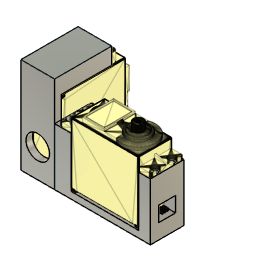
TARO2_arm_upper v1 (Autodesk Fusion 360 design; units mm, degrees)
Autodesk Fusion 360 part; units mm, degrees
sketch "スケッチ1" plane through (0, 0, 0) normal (0, 0, 1) x (1, 0, 0)
  line L0 (0, 0) -> (-34.35, 0)
  line L1 (-34.35, 0) -> (-34.35, 9.85)
  line L2 (-34.35, 9.85) -> (0, 9.85)
  line L3 (0, 9.85) -> (0, 0)
  line L4 (0, 0) -> (-24.35, 0)
  line L5 (-24.35, 0) -> (-24.35, -9.85)
  line L6 (-24.35, -9.85) -> (0, -9.85)
  line L7 (0, -9.85) -> (0, 0)
  line L8 (-34.35, 9.85) -> (14.25, 9.85)
  line L9 (14.25, 9.85) -> (14.25, -10)
  line L10 (14.25, -10) -> (-34.35, -10)
  line L11 (-34.35, -10) -> (-34.35, 9.85)
  line L12 (0, 0) -> (-34.35, 0)
  line L13 (14.25, -10) -> (-34.35, -10)
  line L14 (-34.35, 0) -> (-34.35, 9.85)
  line L15 (14.25, 9.85) -> (14.25, -10)
  line L16 (-34.35, 9.85) -> (14.25, 9.85)
  line L17 (0, 0) -> (-24.35, 0)
  line L18 (0, -9.85) -> (0, 0)
  line L19 (-24.35, 0) -> (-24.35, -9.85)
  line L20 (0, 9.85) -> (0, 0)
  line L21 (-34.35, -10) -> (-34.35, 9.85)
  line L22 (-24.35, -9.85) -> (0, -9.85)
  line L23 (-34.35, 9.85) -> (0, 9.85)
  dimension "d2" = 34.35
  dimension "d3" = 9.85
  dimension "d4" = 9.85
  dimension "d5" = 48.6
  dimension "d6" = 34.35
  dimension "d7" = 9.85
  dimension "d8" = 9.85
  dimension "d9" = 48.6
  constraint horizontal L0
  constraint vertical L1
  constraint horizontal L2
  constraint vertical L3
  constraint horizontal L4
  constraint vertical L5
  constraint horizontal L6
  constraint vertical L7
  constraint horizontal L8
  constraint vertical L9
  constraint horizontal L10
  constraint vertical L11
  constraint horizontal L12
  constraint vertical L14
  constraint horizontal L23
  constraint vertical L20
  constraint horizontal L17
  constraint vertical L19
  constraint horizontal L22
  constraint vertical L18
  constraint horizontal L16
  constraint vertical L15
  constraint horizontal L13
  constraint vertical L21
  measures "d2" distance of L0.start L0.end
  measures "d3" distance of L0.start L2.end
  measures "d4" distance of L0.start L6.end
  measures "d5" distance of L1.end L8.end
  measures "d6" distance of L0.start L0.end
  measures "d7" distance of L0.start L2.end
  measures "d8" distance of L0.start L6.end
  measures "d9" distance of L1.end L8.end
other "基準メッシュ フィーチャ1" in component "MG996R bracket(bairing) v1"
other "修正1" in component "MG996R bracket(bairing) v1"
other "修正2" in component "MG996R bracket(bairing) v1"
sketch "スケッチ1 (2)" plane through (0, 0, 0) normal (0, 0, 1) x (1, 0, 0) in component "MG996R bracket(bairing) v1"
other "修正3" in component "MG996R bracket(bairing) v1"
sketch "スケッチ2" plane through (0, 0, 0) normal (0, 0, 1) x (1, 0, 0) in component "MG996R bracket(bairing) v1"
  line L0 (-20, 10) -> (20, 10)
  line L1 (20, 10) -> (20, -10)
  line L2 (20, -10) -> (-20, -10)
  line L3 (-20, -10) -> (-20, 10)
  line L4 (-20, 10) -> (20, -10) construction
  line L5 (20, 10) -> (-20, -10) construction
  line L6 (20, -10) -> (27, -10)
  line L7 (27, -10) -> (27, 10)
  line L8 (27, 10) -> (20, 10)
  line L9 (20, 10) -> (20, -10)
  line L10 (-20, -10) -> (-27, -10)
  line L11 (-27, -10) -> (-27, 10)
  line L12 (-27, 10) -> (-20, 10)
  line L13 (-20, 10) -> (-20, -10)
  dimension "d1" = 7
  dimension "d2_1" = 20
  dimension "d3_1" = 7
  dimension "d4_1" = 20
  constraint horizontal L0
  constraint perpendicular L0 L1
  constraint parallel L0 L2
  constraint parallel L1 L3
  constraint coincident L4 origin
  constraint coincident L5 origin
  constraint horizontal L6
  constraint vertical L7
  constraint horizontal L8
  constraint vertical L9
  constraint horizontal L10
  constraint vertical L11
  constraint horizontal L12
  constraint vertical L13
  measures "d1" distance of L1.end L6.end
  measures "d2_1" distance of L1.end L0.end
  measures "d3_1" distance of L2.end L10.end
  measures "d4_1" distance of L2.end L0.start
extrude "押し出し1" add sketch "スケッチ2" along normal blind 3 makes body 1 in component "MG996R bracket(bairing) v1"
sketch "スケッチ3" plane through (0, 0, 3) normal (0, 0, 1) x (-1, 0, 0) in component "MG996R bracket(bairing) v1"
  line L0 (27, 10) -> (-27, 10)
  line L1 (-27, 10) -> (-27, -10)
  line L2 (-27, -10) -> (27, -10)
  line L3 (27, -10) -> (27, 10)
  line L4 (27, 10) -> (20, 10)
  line L5 (20, 10) -> (20, -10)
  line L6 (20, -10) -> (27, -10)
  line L7 (27, -10) -> (27, 10)
  line L8 (-27, 10) -> (-20, 10)
  line L9 (-20, 10) -> (-20, -10)
  line L10 (-20, -10) -> (-27, -10)
  line L11 (-27, -10) -> (-27, 10)
  constraint horizontal L4
  constraint vertical L5
  constraint horizontal L6
  constraint vertical L7
  constraint coincident L2 L5.end
  constraint coincident L0.start L3.end
  constraint horizontal L8
  constraint vertical L9
  constraint horizontal L10
  constraint vertical L11
  constraint coincident L0.end L1.start
extrude "押し出し2" add sketch "スケッチ3" along normal blind 5 contours L0 L2 L3 L4 L5 L6 L7 | L0 L1 L2 L8 L9 L10 L11 bodies 1 in component "MG996R bracket(bairing) v1"
sketch "スケッチ4" plane through (0, 0, 8) normal (0, 0, 1) x (-1, 0, 0) in component "MG996R bracket(bairing) v1"
  line L0 (-27, -10) -> (-20, -10)
  line L1 (-20, -10) -> (-20, 10)
  line L2 (-20, 10) -> (-27, 10)
  line L3 (-27, 10) -> (-27, -10)
  line L4 (-20, 10) -> (-27, 10)
  line L5 (-27, 10) -> (-27, 5)
  line L6 (-27, 5) -> (-20, 5)
  line L7 (-20, 5) -> (-20, 10)
  line L8 (-27, -10) -> (-20, -10)
  line L9 (-20, -10) -> (-20, -5)
  line L10 (-20, -5) -> (-27, -5)
  line L11 (-27, -5) -> (-27, -10)
  dimension "d9_1" = 7
  dimension "d10" = 5
  constraint horizontal L4
  constraint vertical L5
  constraint horizontal L6
  constraint vertical L7
  constraint coincident L3 L5.end
  constraint coincident L1.end L2.start
  constraint horizontal L8
  constraint vertical L9
  constraint horizontal L10
  constraint vertical L11
  constraint coincident L0.start L3.end
  measures "d9_1" distance of L0.start L0.end
  measures "d10" distance of L0.start L10.end
extrude "押し出し3" add sketch "スケッチ4" along normal blind 9 contours L0 L1 L3 L8 L9 L10 L11 | L1 L2 L3 L4 L5 L6 L7 bodies 1 in component "MG996R bracket(bairing) v1"
sketch "スケッチ5" plane through (0, 0, 17) normal (0, 0, 1) x (-1, 0, 0) in component "MG996R bracket(bairing) v1"
  line L0 (-27, -5) -> (-27, -10)
  line L1 (-27, -10) -> (-20, -10)
  line L2 (-20, -10) -> (-20, -5)
  line L3 (-20, -5) -> (-27, -5)
  line L4 (-20, 10) -> (-27, 10)
  line L5 (-27, 10) -> (-27, -10)
  line L6 (-27, -10) -> (-20, -10)
  line L7 (-20, -10) -> (-20, 10)
  constraint horizontal L4
  constraint vertical L5
  constraint horizontal L6
  constraint vertical L7
  constraint coincident L0.end L1.start
extrude "押し出し4" add sketch "スケッチ5" along normal blind 16 bodies 1 in component "MG996R bracket(bairing) v1"
extrude "押し出し5" add 1 faces at (-22.3333, 3.3333, 8) along direction (0, 0, 1) blind 25 on bodies 1 bodies 1 in component "MG996R bracket(bairing) v1"
sketch "スケッチ6" plane through (0, 0, 33) normal (0, 0, 1) x (-1, 0, 0) in component "MG996R bracket(bairing) v1"
  line L0 (-20, -10) -> (-20, 10)
  line L1 (-20, 10) -> (-27, 10)
  line L2 (-27, 10) -> (-27, -10)
  line L3 (-27, -10) -> (-20, -10)
  circle A0 centre (-25, 5) radius 1.5
  circle A1 centre (-25, -5) radius 1.5
  circle A2 centre (24.95, 5.2) radius 1.5
  circle A3 centre (25, -4.8) radius 1.5
  dimension "d17" = 3
  dimension "d18" = 3
  dimension "d19" = 3
  dimension "d20" = 3
  measures "d17" diameter of A0
  measures "d18" diameter of A1
  measures "d19" diameter of A2
  measures "d20" diameter of A3
extrude "押し出し6" cut sketch "スケッチ6" against normal blind 5 contours A0 | A1 | A2 | A3 bodies 1 in component "MG996R bracket(bairing) v1"
thread "ねじ1" "ISO Metric profile 3.0 M3x0.5 M3x0.5 6H" major diameter 3.086 minor diameter 2.529 pitch 0.5 angle 60 resizes the face on face at (-26.4981, 4.8748, 29.6667) on bodies 1 in component "MG996R bracket(bairing) v1"
thread "ねじ2" "ISO Metric profile 3.0 M3x0.5 M3x0.5 6H" major diameter 3.086 minor diameter 2.529 pitch 0.5 angle 60 resizes the face on face at (-26.4481, -5.1252, 29.6667) on bodies 1 in component "MG996R bracket(bairing) v1"
thread "ねじ3" "ISO Metric profile 3.0 M3x0.5 M3x0.5 6H" major diameter 3.086 minor diameter 2.529 pitch 0.5 angle 60 resizes the face on face at (23.5019, -4.9252, 29.6667) on face at (23.5019, 5.0748, 29.6667) on bodies 1 in component "MG996R bracket(bairing) v1"
extrude "押し出し7" add 1 faces at (-9, -3.3333, 0) along direction (0, 0, -1) blind 1 on bodies 1 bodies 1 in component "MG996R bracket(bairing) v1"
sketch "スケッチ7" plane through (0, 0, 0) normal (0, 0, 1) x (1, 0, 0) in component "MG996R bracket(bairing) v1"
  line L0 (-20, -10) -> (10.1, -10)
  line L1 (10.1, -10) -> (10.1, 10)
  line L2 (10.1, 10) -> (-20, 10)
  line L3 (-20, 10) -> (-20, -10)
  circle A0 centre (10.1, 0) radius 7
  dimension "d31" = 30.1
  dimension "d32" = 14
  constraint horizontal L0
  constraint vertical L1
  constraint horizontal L2
  constraint vertical L3
  constraint midpoint L1 A0.centre
  measures "d31" distance of L0.start L0.end
  measures "d32" diameter of A0
move_body "移動1" bodies 1 to x (1, 0, 0) y (0, 1, 0) z (0, 0, 1) at (0, 0, 1) in component "MG996R bracket(bairing) v1"
other "修正4" in component "MG996R bracket(bairing) v1"
extrude "押し出し8" cut sketch "スケッチ7" along normal blind 4 contours L1 A0 | L1 A0 bodies 1 in component "MG996R bracket(bairing) v1"
extrude "押し出し9" add 1 faces at (-27, -3.3333, 11.3333) along direction (-1, 0, 0) blind 3 on bodies 1 bodies 1 in component "MG996R bracket(bairing) v1"
sketch "スケッチ8" plane through (-30, 0, 0) normal (-1, 0, 0) x (0, -1, 0) in component "MG996R bracket(bairing) v1"
  line L0 (10, 0) -> (10, 34)
  line L1 (10, 34) -> (-10, 34)
  line L2 (-10, 34) -> (-10, 0)
  line L3 (-10, 0) -> (10, 0)
other "基準メッシュ フィーチャ1'" in component "MG996R bracket(bairing) v1 (1)"
other "修正1'" in component "MG996R bracket(bairing) v1 (1)"
other "修正2'" in component "MG996R bracket(bairing) v1 (1)"
sketch "スケッチ1 (3)" plane through (0, 0, 0) normal (0, 0, 1) x (1, 0, 0) in component "MG996R bracket(bairing) v1 (1)"
other "修正3'" in component "MG996R bracket(bairing) v1 (1)"
sketch "スケッチ2 (2)" plane through (0, 0, 0) normal (0, 0, 1) x (1, 0, 0) in component "MG996R bracket(bairing) v1 (1)"
  line L0 (-20, 10) -> (20, 10)
  line L1 (20, 10) -> (20, -10)
  line L2 (20, -10) -> (-20, -10)
  line L3 (-20, -10) -> (-20, 10)
  line L4 (-20, 10) -> (20, -10) construction
  line L5 (20, 10) -> (-20, -10) construction
  line L6 (20, -10) -> (27, -10)
  line L7 (27, -10) -> (27, 10)
  line L8 (27, 10) -> (20, 10)
  line L9 (20, 10) -> (20, -10)
  line L10 (-20, -10) -> (-27, -10)
  line L11 (-27, -10) -> (-27, 10)
  line L12 (-27, 10) -> (-20, 10)
  line L13 (-20, 10) -> (-20, -10)
  dimension "d1_1" = 7
  dimension "d2_2" = 20
  dimension "d3_2" = 7
  dimension "d4_2" = 20
  constraint horizontal L0
  constraint perpendicular L0 L1
  constraint parallel L0 L2
  constraint parallel L1 L3
  constraint coincident L4 origin
  constraint coincident L5 origin
  constraint horizontal L6
  constraint vertical L7
  constraint horizontal L8
  constraint vertical L9
  constraint horizontal L10
  constraint vertical L11
  constraint horizontal L12
  constraint vertical L13
  measures "d1_1" distance of L1.end L6.end
  measures "d2_2" distance of L1.end L0.end
  measures "d3_2" distance of L2.end L10.end
  measures "d4_2" distance of L2.end L0.start
extrude "押し出し1'" add sketch "スケッチ2 (2)" along normal blind 3 separate body makes body 2 in component "MG996R bracket(bairing) v1 (1)"
sketch "スケッチ3 (2)" plane through (0, 0, 3) normal (0, 0, 1) x (-1, 0, 0) in component "MG996R bracket(bairing) v1 (1)"
  line L0 (27, 10) -> (-27, 10)
  line L1 (-27, 10) -> (-27, -10)
  line L2 (-27, -10) -> (27, -10)
  line L3 (27, -10) -> (27, 10)
  line L4 (27, 10) -> (20, 10)
  line L5 (20, 10) -> (20, -10)
  line L6 (20, -10) -> (27, -10)
  line L7 (27, -10) -> (27, 10)
  line L8 (-27, 10) -> (-20, 10)
  line L9 (-20, 10) -> (-20, -10)
  line L10 (-20, -10) -> (-27, -10)
  line L11 (-27, -10) -> (-27, 10)
  constraint horizontal L4
  constraint vertical L5
  constraint horizontal L6
  constraint vertical L7
  constraint coincident L2 L5.end
  constraint coincident L0.start L3.end
  constraint horizontal L8
  constraint vertical L9
  constraint horizontal L10
  constraint vertical L11
  constraint coincident L0.end L1.start
extrude "押し出し2'" add sketch "スケッチ3 (2)" along normal blind 5 contours L0 L2 L3 L4 L5 L6 L7 | L0 L1 L2 L8 L9 L10 L11 bodies 2 in component "MG996R bracket(bairing) v1 (1)"
sketch "スケッチ4 (2)" plane through (0, 0, 8) normal (0, 0, 1) x (-1, 0, 0) in component "MG996R bracket(bairing) v1 (1)"
  line L0 (-27, -10) -> (-20, -10)
  line L1 (-20, -10) -> (-20, 10)
  line L2 (-20, 10) -> (-27, 10)
  line L3 (-27, 10) -> (-27, -10)
  line L4 (-20, 10) -> (-27, 10)
  line L5 (-27, 10) -> (-27, 5)
  line L6 (-27, 5) -> (-20, 5)
  line L7 (-20, 5) -> (-20, 10)
  line L8 (-27, -10) -> (-20, -10)
  line L9 (-20, -10) -> (-20, -5)
  line L10 (-20, -5) -> (-27, -5)
  line L11 (-27, -5) -> (-27, -10)
  dimension "d9_2" = 7
  dimension "d10_1" = 5
  constraint horizontal L4
  constraint vertical L5
  constraint horizontal L6
  constraint vertical L7
  constraint coincident L3 L5.end
  constraint coincident L1.end L2.start
  constraint horizontal L8
  constraint vertical L9
  constraint horizontal L10
  constraint vertical L11
  constraint coincident L0.start L3.end
  measures "d9_2" distance of L0.start L0.end
  measures "d10_1" distance of L0.start L10.end
extrude "押し出し3'" add sketch "スケッチ4 (2)" along normal blind 9 contours L0 L1 L3 L8 L9 L10 L11 | L1 L2 L3 L4 L5 L6 L7 bodies 2 in component "MG996R bracket(bairing) v1 (1)"
sketch "スケッチ5 (2)" plane through (0, 0, 17) normal (0, 0, 1) x (-1, 0, 0) in component "MG996R bracket(bairing) v1 (1)"
  line L0 (-27, -5) -> (-27, -10)
  line L1 (-27, -10) -> (-20, -10)
  line L2 (-20, -10) -> (-20, -5)
  line L3 (-20, -5) -> (-27, -5)
  line L4 (-20, 10) -> (-27, 10)
  line L5 (-27, 10) -> (-27, -10)
  line L6 (-27, -10) -> (-20, -10)
  line L7 (-20, -10) -> (-20, 10)
  constraint horizontal L4
  constraint vertical L5
  constraint horizontal L6
  constraint vertical L7
  constraint coincident L0.end L1.start
extrude "押し出し4'" add sketch "スケッチ5 (2)" along normal blind 16 bodies 2 in component "MG996R bracket(bairing) v1 (1)"
extrude "押し出し5'" add 1 faces at (-22.3333, 3.3333, 8) along direction (0, 0, 1) blind 25 on bodies 2 bodies 2 in component "MG996R bracket(bairing) v1 (1)"
sketch "スケッチ6 (2)" plane through (0, 0, 33) normal (0, 0, 1) x (-1, 0, 0) in component "MG996R bracket(bairing) v1 (1)"
  line L0 (-20, -10) -> (-20, 10)
  line L1 (-20, 10) -> (-27, 10)
  line L2 (-27, 10) -> (-27, -10)
  line L3 (-27, -10) -> (-20, -10)
  circle A0 centre (-25, 5) radius 1.5
  circle A1 centre (-25, -5) radius 1.5
  circle A2 centre (24.95, 5.2) radius 1.5
  circle A3 centre (25, -4.8) radius 1.5
  dimension "d17_1" = 3
  dimension "d18_1" = 3
  dimension "d19_1" = 3
  dimension "d20_1" = 3
  measures "d17_1" diameter of A0
  measures "d18_1" diameter of A1
  measures "d19_1" diameter of A2
  measures "d20_1" diameter of A3
extrude "押し出し6'" cut sketch "スケッチ6 (2)" against normal blind 5 contours A0 | A1 | A2 | A3 bodies 2 in component "MG996R bracket(bairing) v1 (1)"
thread "ねじ1'" "ISO Metric profile 3.0 M3x0.5 M3x0.5 6H" major diameter 3.086 minor diameter 2.529 pitch 0.5 angle 60 resizes the face on face at (-26.4981, 4.8748, 29.6667) on bodies 2 in component "MG996R bracket(bairing) v1 (1)"
thread "ねじ2'" "ISO Metric profile 3.0 M3x0.5 M3x0.5 6H" major diameter 3.086 minor diameter 2.529 pitch 0.5 angle 60 resizes the face on face at (-26.4481, -5.1252, 29.6667) on bodies 2 in component "MG996R bracket(bairing) v1 (1)"
thread "ねじ3'" "ISO Metric profile 3.0 M3x0.5 M3x0.5 6H" major diameter 3.086 minor diameter 2.529 pitch 0.5 angle 60 resizes the face on face at (23.5019, -4.9252, 29.6667) on face at (23.5019, 5.0748, 29.6667) on bodies 2 in component "MG996R bracket(bairing) v1 (1)"
extrude "押し出し7'" add 1 faces at (-9, -3.3333, 0) along direction (0, 0, -1) blind 1 on bodies 2 bodies 2 in component "MG996R bracket(bairing) v1 (1)"
sketch "スケッチ7 (2)" plane through (0, 0, 0) normal (0, 0, 1) x (1, 0, 0) in component "MG996R bracket(bairing) v1 (1)"
  line L0 (-20, -10) -> (10.1, -10)
  line L1 (10.1, -10) -> (10.1, 10)
  line L2 (10.1, 10) -> (-20, 10)
  line L3 (-20, 10) -> (-20, -10)
  circle A0 centre (10.1, 0) radius 7
  dimension "d31_1" = 30.1
  dimension "d32_1" = 14
  constraint horizontal L0
  constraint vertical L1
  constraint horizontal L2
  constraint vertical L3
  constraint midpoint L1 A0.centre
  measures "d31_1" distance of L0.start L0.end
  measures "d32_1" diameter of A0
move_body "移動1'" bodies 2 to x (1, 0, 0) y (0, 1, 0) z (0, 0, 1) at (0, 0, 1) in component "MG996R bracket(bairing) v1 (1)"
other "修正4'" in component "MG996R bracket(bairing) v1 (1)"
extrude "押し出し8'" cut sketch "スケッチ7 (2)" along normal blind 4 contours L1 A0 | L1 A0 bodies 2 in component "MG996R bracket(bairing) v1 (1)"
extrude "押し出し9'" add 1 faces at (-27, -3.3333, 11.3333) along direction (-1, 0, 0) blind 3 on bodies 2 bodies 2 in component "MG996R bracket(bairing) v1 (1)"
sketch "スケッチ8 (2)" plane through (-30, 0, 0) normal (-1, 0, 0) x (0, -1, 0) in component "MG996R bracket(bairing) v1 (1)"
  line L0 (10, 0) -> (10, 34)
  line L1 (10, 34) -> (-10, 34)
  line L2 (-10, 34) -> (-10, 0)
  line L3 (-10, 0) -> (10, 0)
combine "結合1" operation add target body 2 tool bodies 1 body 1 seen with x (0, -1, 0) y (0, 0, 1) z (-1, 0, 0) at (27.0001, -40, 9.9999) in component "MG996R bracket(bairing) v1 (1)"
component "MG996R bracket(bairing) v1" placed x (1, 0, 0) y (0, 1, 0) z (0, 0, 1) at (0, 0, 0)
component "MG996R bracket(bairing) v1 (1)" placed x (0, 0, -1) y (-1, 0, 0) z (0, 1, 0) at (-40, -9.9999, 27.0001)
